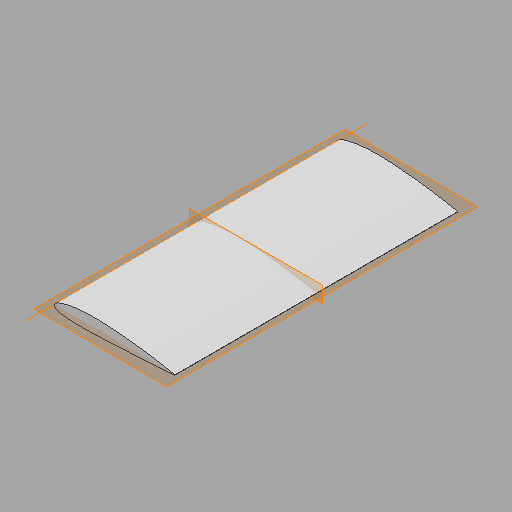
# Autodesk Inventor part: MiddleWing
Saved by Autodesk Inventor 2025 (Build 290162000, 162)
## iProperties
Created: 2025-06-04
Part Number: MiddleWing
Material: Generic
Document SubType Name: Modeling
Designer: Cupri
Density: 1 g/cm^3
Appearance: Default
Author: Cupri
Autodesk Inventor part; units mm, degrees
ref_plane "YZ Plane" through (0, 0, 0) normal (1, 0, 0) x (0, 1, 0)
ref_plane "XZ Plane" through (0, 0, 0) normal (0, 1, 0) x (-1, 0, 0)
ref_plane "XY Plane" through (0, 0, 0) normal (0, 0, 1) x (1, 0, 0)
sketch "Sketch1" plane through (0, 0, 0) normal (0, 0, 1) x (1, 0, 0)
  spline S0 degree 4 poles (320.0269, 0.4022) (319.9788, 0.4121) (319.7452, 0.4612) (319.3526, 0.5426) (318.6898, 0.6806) (317.9926, 0.8246) (317.136, 1.0019) (316.1274, 1.2091) (314.9648, 1.4466) (313.6506, 1.714) (312.1859, 2.0099) (310.5719, 2.3346) (308.8099, 2.6849) (306.9023, 3.0623) (304.8502, 3.464) (302.6559, 3.8904) (300.3211, 4.3383) (297.8485, 4.8089) (295.2403, 5.2983) (292.4983, 5.8079) (289.626, 6.334) (286.6256, 6.8769) (283.5002, 7.4342) (280.2525, 8.0051) (276.886, 8.588) (273.4032, 9.1804) (269.8085, 9.7837) (266.1043, 10.3926) (262.2951, 11.0088) (258.3838, 11.6297) (254.3743, 12.253) (250.2709, 12.8789) (246.0772, 13.5044) (241.7974, 14.1284) (237.436, 14.7509) (232.9961, 15.3683) (228.4838, 15.98) (223.9017, 16.5854) (219.2555, 17.1817) (214.5494, 17.7686) (209.788, 18.3433) (204.9761, 18.9063) (200.1181, 19.4542) (195.2192, 19.9873) (190.2842, 20.5034) (185.3173, 21.0005) (180.3249, 21.4788) (175.3103, 21.9353) (170.2797, 22.3705) (165.2375, 22.781) (160.189, 23.1672) (155.1389, 23.5278) (150.0934, 23.8603) (145.0556, 24.1654) (140.0323, 24.44) (135.0234, 24.6851) (130.0426, 24.8979) (125.067, 25.0797) (120.1128, 25.214) (115.1972, 25.3059) (110.3234, 25.3527) (105.4982, 25.3539) (100.7275, 25.3101) (96.0158, 25.2215) (91.3687, 25.0871) (86.791, 24.9082) (82.2872, 24.6849) (77.8623, 24.4175) (73.521, 24.1062) (69.2675, 23.7535) (65.1072, 23.358) (61.0435, 22.9232) (57.0814, 22.4481) (53.2243, 21.9351) (49.4771, 21.3859) (45.8428, 20.8014) (42.3261, 20.1835) (38.9297, 19.5335) (35.6574, 18.8535) (32.5127, 18.1458) (29.4984, 17.411) (26.6175, 16.6531) (23.8731, 15.872) (21.2678, 15.0705) (18.8035, 14.2514) (16.4833, 13.4153) (14.3089, 12.5652) (12.2822, 11.7027) (10.4049, 10.8295) (8.6792, 9.9473) (7.1054, 9.0582) (5.6853, 8.1638) (4.4202, 7.2643) (3.3093, 6.3629) (2.3554, 5.4578) (1.5572, 4.5511) (0.9163, 3.6427) (0.4341, 2.7315) (0.1142, 1.818) (-0.0431, 0.9059) (-0.0334, -0.0033) (0.1374, -0.8964) (0.4711, -1.7593) (0.9639, -2.5913) (1.6124, -3.39) (2.414, -4.1565) (3.3664, -4.8908) (4.4685, -5.5951) (5.719, -6.2694) (7.117, -6.914) (8.6612, -7.5288) (10.35, -8.1136) (12.182, -8.6687) (14.155, -9.1934) (16.2675, -9.6882) (18.5167, -10.1522) (20.9012, -10.5863) (23.4176, -10.99) (26.0643, -11.362) (28.8379, -11.7053) (31.7363, -12.017) (34.756, -12.2994) (37.8948, -12.5514) (41.1489, -12.7743) (44.5156, -12.9683) (47.992, -13.1332) (51.574, -13.2706) (55.2589, -13.3808) (59.0428, -13.4647) (62.9227, -13.5221) (66.8947, -13.5562) (70.9548, -13.5656) (75.1003, -13.5526) (79.326, -13.5183) (83.6294, -13.4632) (88.0056, -13.3897) (92.4508, -13.298) (96.9617, -13.1901) (101.5332, -13.0674) (106.1614, -12.9303) (110.8425, -12.7826) (115.5719, -12.6221) (120.3483, -12.4545) (125.1641, -12.276) (130.0277, -12.0954) (134.9445, -11.8975) (139.8831, -11.6864) (144.8465, -11.461) (149.8259, -11.2244) (154.8163, -10.9762) (159.8128, -10.7197) (164.8106, -10.4534) (169.8048, -10.1803) (174.7908, -9.9005) (179.7633, -9.6155) (184.7174, -9.3259) (189.6491, -9.0328) (194.5523, -8.7371) (199.4236, -8.4398) (204.2568, -8.1406) (209.0483, -7.8424) (213.7927, -7.543) (218.4853, -7.246) (223.1219, -6.9495) (227.6975, -6.6557) (232.2074, -6.3642) (236.6478, -6.0762) (241.0133, -5.7913) (245.3008, -5.511) (249.5045, -5.2345) (253.6216, -4.963) (257.6469, -4.6967) (261.5771, -4.4354) (265.4075, -4.1795) (269.1353, -3.931) (272.7553, -3.6871) (276.2653, -3.4506) (279.6605, -3.2209) (282.9381, -2.9986) (286.0948, -2.7826) (289.1271, -2.5755) (292.0318, -2.3754) (294.8063, -2.1837) (297.4477, -2.0012) (299.9529, -1.8261) (302.3195, -1.6611) (304.5456, -1.5046) (306.6278, -1.3576) (308.565, -1.2212) (310.3547, -1.0934) (311.9949, -0.977) (313.4842, -0.8705) (314.8207, -0.7744) (316.0035, -0.6897) (317.0298, -0.6151) (317.9019, -0.5528) (318.6116, -0.5011) (319.2867, -0.4521) (319.686, -0.4236) (319.9244, -0.4056) (319.9731, -0.4022) knots 0 0 0 0 0 0.003306 0.005253 0.007519 0.010061 0.012848 0.015859 0.019076 0.022485 0.026074 0.029832 0.033751 0.037822 0.042038 0.046391 0.050876 0.055485 0.060215 0.065059 0.070013 0.075071 0.08023 0.085484 0.090829 0.096262 0.101778 0.107373 0.113043 0.118786 0.124596 0.13047 0.136405 0.142397 0.148443 0.15454 0.160683 0.16687 0.173096 0.17936 0.185657 0.191984 0.198338 0.204716 0.211115 0.21753 0.22396 0.230401 0.236849 0.243301 0.249755 0.256206 0.262653 0.269091 0.275517 0.281933 0.288337 0.294726 0.301098 0.307445 0.313761 0.320043 0.326289 0.332494 0.338655 0.34477 0.350834 0.356845 0.362799 0.368693 0.374523 0.380287 0.38598 0.391599 0.39714 0.402601 0.407977 0.413264 0.41846 0.423559 0.428559 0.433456 0.438244 0.442921 0.447482 0.451924 0.456241 0.46043 0.464487 0.468409 0.472191 0.475831 0.479328 0.482682 0.485897 0.488977 0.491938 0.494796 0.49758 0.500318 0.50304 0.505778 0.508561 0.511418 0.514375 0.51745 0.520657 0.524001 0.527485 0.531109 0.534872 0.53877 0.5428 0.546959 0.551243 0.555647 0.560167 0.5648 0.56954 0.574385 0.57933 0.584371 0.589505 0.594728 0.600036 0.605426 0.610894 0.616437 0.622051 0.627734 0.633481 0.63929 0.645158 0.651081 0.657056 0.66308 0.66915 0.675263 0.681415 0.687604 0.693827 0.700081 0.706365 0.71268 0.719023 0.72539 0.731777 0.738175 0.744583 0.750996 0.757412 0.763827 0.770239 0.776645 0.78304 0.789422 0.795788 0.802134 0.808458 0.814756 0.821025 0.827261 0.833462 0.839624 0.845743 0.851817 0.857841 0.863813 0.869729 0.875585 0.881378 0.887104 0.892759 0.898341 0.903844 0.909264 0.914599 0.919843 0.924992 0.930042 0.934988 0.939826 0.944549 0.949154 0.953634 0.957983 0.962194 0.966262 0.970179 0.973935 0.977522 0.98093 0.984146 0.987156 0.989942 0.992483 0.994749 0.996695 1 1 1 1 1
  arc A0 (319.9731, -0.4022) -> (320.0269, 0.4022) centre (319.8668, 0.0089) ccw
  line L0 (0, 0) -> (320.2905, -0.0194)
  point P0 (319.9485, 0.4186)
  point P1 (319.7139, 0.4675)
  point P2 (319.3232, 0.5488)
  point P3 (318.7766, 0.6624)
  point P4 (318.0749, 0.8077)
  point P5 (317.2182, 0.9846)
  point P6 (316.208, 1.1923)
  point P7 (315.0448, 1.4301)
  point P8 (313.7296, 1.6976)
  point P9 (312.264, 1.9939)
  point P10 (310.649, 2.3184)
  point P11 (308.8861, 2.6694)
  point P12 (306.9773, 3.0467)
  point P13 (304.9242, 3.449)
  point P14 (302.7286, 3.8752)
  point P15 (300.3926, 4.3238)
  point P16 (297.9187, 4.7942)
  point P17 (295.3091, 5.2845)
  point P18 (292.5658, 5.7939)
  point P19 (289.6918, 6.3206)
  point P20 (286.6899, 6.8637)
  point P21 (283.5629, 7.4214)
  point P22 (280.3136, 7.9926)
  point P23 (276.9453, 8.5757)
  point P24 (273.4608, 9.169)
  point P25 (269.864, 9.7718)
  point P26 (266.1581, 10.3818)
  point P27 (262.3469, 10.9981)
  point P28 (258.4336, 11.6192)
  point P29 (254.4221, 12.2432)
  point P30 (250.3165, 12.8691)
  point P31 (246.1206, 13.495)
  point P32 (241.8387, 14.1197)
  point P33 (237.4749, 14.7421)
  point P34 (233.033, 15.36)
  point P35 (228.5181, 15.9722)
  point P36 (223.9338, 16.5776)
  point P37 (219.2851, 17.1744)
  point P38 (214.5766, 17.7613)
  point P39 (209.8128, 18.3366)
  point P40 (204.9984, 18.8995)
  point P41 (200.1379, 19.448)
  point P42 (195.2365, 19.9811)
  point P43 (190.2989, 20.4973)
  point P44 (185.3296, 20.9949)
  point P45 (180.3344, 21.473)
  point P46 (175.3174, 21.9299)
  point P47 (170.2842, 22.3648)
  point P48 (165.2394, 22.7757)
  point P49 (160.1882, 23.1619)
  point P50 (155.1357, 23.5222)
  point P51 (150.0874, 23.855)
  point P52 (145.0474, 24.1597)
  point P53 (140.0214, 24.4346)
  point P54 (135.0147, 24.679)
  point P55 (130.032, 24.8918)
  point P56 (125.0547, 25.0704)
  point P57 (120.095, 25.2058)
  point P58 (115.1741, 25.297)
  point P59 (110.2976, 25.3434)
  point P60 (105.4701, 25.3443)
  point P61 (100.697, 25.3002)
  point P62 (95.983, 25.2109)
  point P63 (91.3338, 25.0762)
  point P64 (86.7539, 24.8966)
  point P65 (82.248, 24.6726)
  point P66 (77.8211, 24.4045)
  point P67 (73.4778, 24.0928)
  point P68 (69.2224, 23.7389)
  point P69 (65.0602, 23.343)
  point P70 (60.9949, 22.9069)
  point P71 (57.031, 22.431)
  point P72 (53.1725, 21.9171)
  point P73 (49.4237, 21.3667)
  point P74 (45.7882, 20.7811)
  point P75 (42.2701, 20.1619)
  point P76 (38.8726, 19.5107)
  point P77 (35.5994, 18.8294)
  point P78 (32.4538, 18.12)
  point P79 (29.4387, 17.384)
  point P80 (26.5574, 16.624)
  point P81 (23.8128, 15.8413)
  point P82 (21.2074, 15.0381)
  point P83 (18.7434, 14.2166)
  point P84 (16.4237, 13.3786)
  point P85 (14.2502, 12.5261)
  point P86 (12.225, 11.6611)
  point P87 (10.3498, 10.7853)
  point P88 (8.6266, 9.9005)
  point P89 (7.0563, 9.0086)
  point P90 (5.641, 8.1114)
  point P91 (4.3814, 7.2099)
  point P92 (3.2784, 6.3062)
  point P93 (2.3334, 5.401)
  point P94 (1.5466, 4.4957)
  point P95 (0.9184, 3.5917)
  point P96 (0.4496, 2.6893)
  point P97 (0.1405, 1.7894)
  point P98 (-0.0096, 0.8928)
  point P99 (0.1674, -0.8771)
  point P100 (0.4912, -1.7264)
  point P101 (0.9706, -2.5475)
  point P102 (1.6048, -3.3405)
  point P103 (2.3933, -4.105)
  point P104 (3.3347, -4.8403)
  point P105 (4.4282, -5.5469)
  point P106 (5.672, -6.2243)
  point P107 (7.065, -6.8723)
  point P108 (8.6054, -7.4906)
  point P109 (10.2915, -8.0787)
  point P110 (12.1216, -8.6368)
  point P111 (14.0934, -9.1645)
  point P112 (16.2051, -9.6618)
  point P113 (18.4541, -10.1283)
  point P114 (20.8384, -10.5645)
  point P115 (23.3552, -10.9699)
  point P116 (26.0022, -11.3443)
  point P117 (28.7766, -11.6886)
  point P118 (31.6758, -12.0022)
  point P119 (34.6966, -12.2858)
  point P120 (37.8365, -12.5392)
  point P121 (41.0918, -12.7632)
  point P122 (44.4598, -12.9581)
  point P123 (47.9376, -13.1242)
  point P124 (51.5213, -13.2624)
  point P125 (55.2077, -13.3734)
  point P126 (58.9933, -13.4579)
  point P127 (62.8749, -13.5165)
  point P128 (66.8486, -13.5507)
  point P129 (70.9107, -13.561)
  point P130 (75.0579, -13.5485)
  point P131 (79.2858, -13.5146)
  point P132 (83.591, -13.4602)
  point P133 (87.9693, -13.3869)
  point P134 (92.4166, -13.2957)
  point P135 (96.9296, -13.1882)
  point P136 (101.5034, -13.0656)
  point P137 (106.1338, -12.9293)
  point P138 (110.817, -12.7811)
  point P139 (115.5485, -12.6218)
  point P140 (120.3242, -12.4534)
  point P141 (125.1395, -12.2768)
  point P142 (130.0061, -12.0931)
  point P143 (134.9261, -11.8957)
  point P144 (139.8717, -11.6842)
  point P145 (144.8378, -11.4592)
  point P146 (149.8198, -11.2224)
  point P147 (154.8128, -10.9747)
  point P148 (159.8118, -10.7178)
  point P149 (164.8122, -10.4518)
  point P150 (169.809, -10.1786)
  point P151 (174.7974, -9.8989)
  point P152 (179.7725, -9.6138)
  point P153 (184.7293, -9.3242)
  point P154 (189.6634, -9.031)
  point P155 (194.5693, -8.7354)
  point P156 (199.4429, -8.4378)
  point P157 (204.2787, -8.1389)
  point P158 (209.0726, -7.84)
  point P159 (213.8195, -7.5411)
  point P160 (218.5146, -7.2435)
  point P161 (223.1536, -6.9472)
  point P162 (227.7315, -6.6531)
  point P163 (232.2438, -6.3616)
  point P164 (236.6864, -6.0733)
  point P165 (241.0544, -5.7885)
  point P166 (245.344, -5.5078)
  point P167 (249.5501, -5.2314)
  point P168 (253.6691, -4.9597)
  point P169 (257.6966, -4.6931)
  point P170 (261.6288, -4.4317)
  point P171 (265.4614, -4.176)
  point P172 (269.191, -3.9267)
  point P173 (272.8131, -3.6832)
  point P174 (276.3248, -3.4464)
  point P175 (279.7219, -3.2166)
  point P176 (283.0013, -2.9939)
  point P177 (286.1597, -2.7782)
  point P178 (289.1936, -2.5706)
  point P179 (292.0998, -2.3706)
  point P180 (294.8758, -2.1789)
  point P181 (297.5187, -1.9958)
  point P182 (300.0253, -1.8211)
  point P183 (302.3933, -1.6557)
  point P184 (304.6205, -1.4992)
  point P185 (306.704, -1.3523)
  point P186 (308.6422, -1.2154)
  point P187 (310.433, -1.088)
  point P188 (312.0742, -0.9712)
  point P189 (313.5645, -0.8646)
  point P190 (314.9021, -0.7686)
  point P191 (316.0854, -0.6835)
  point P192 (317.1136, -0.6093)
  point P193 (317.9856, -0.5466)
  point P194 (318.7002, -0.4947)
  point P195 (319.2566, -0.4544)
  point P196 (319.6544, -0.4256)
  point P197 (319.8934, -0.408)
  constraints: 3 point on circle, 2 end point, 1 centre point, 201 other
extrude "Extrusion1" add sketch "Sketch1" along normal mid plane 750
ref_plane "Work Plane1" through (0.299, 2.3071, -375) normal (0.0059578, 0.9999823, 0) x (0, 0, 1)
ref_plane "Work Plane2" through (0, 0, 0) normal (0, 0, 1) x (1, 0, 0)
body "Solid1"
